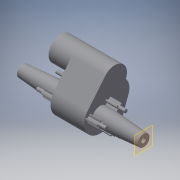
# Autodesk Inventor part: Back_Wheel_Drive
Saved by Autodesk Inventor 2019 (Build 230136000, 136)
## iProperties
Created: 2019-03-02
Part Number: Back_Wheel_Drive
Material: Generic
Document SubType Name: Modeling
Designer: alarr
Density: 1 g/cm^3
Appearance: Default
Author: alarr
Autodesk Inventor part; units mm, degrees
ref_plane "YZ Plane" through (0, 0, 0) normal (1, 0, 0) x (0, 1, 0)
ref_plane "XZ Plane" through (0, 0, 0) normal (0, 1, 0) x (-1, 0, 0)
ref_plane "XY Plane" through (0, 0, 0) normal (0, 0, 1) x (1, 0, 0)
sketch "Sketch1" plane through (0, 0, 0) normal (1, 0, 0) x (0, 1, 0)
  arc A0 (24.2941, -15.0442) -> (28.3956, -3.1971) centre (0, 0) ccw construction
  arc A1 (33.6079, -46.4865) -> (56.8822, -9.6036) centre (42.9735, -26.6116) ccw
  line L0 (18.0894, 22.1202) -> (56.8822, -9.6036)
  line L1 (-28.575, 0) -> (-28.575, -38.1)
  line L2 (-28.575, -38.1) -> (7.1559, -51.3254)
  arc A2 (-10.0486, -26.7499) -> (7.1559, -51.3254) centre (16.3035, -26.6116) ccw construction
  line L3 (42.9735, -26.6116) -> (16.3035, -26.6116) construction
  arc A3 (21.0025, -26.6116) -> (33.6079, -46.4865) centre (42.9735, -26.6116) ccw construction
  arc A4 (-10.0486, -26.7499) -> (24.2941, -15.0442) centre (0, 0) ccw construction
  arc A5 (28.3956, -3.1971) -> (18.0894, 22.1202) centre (0, 0) ccw construction
  arc A6 (18.0894, 22.1202) -> (-28.575, 0) centre (0, 0) ccw
  arc A7 (56.8822, -9.6036) -> (21.0025, -26.6116) centre (42.9735, -26.6116) ccw construction
  arc A8 (28.3956, -3.1971) -> (-10.0486, -26.7499) centre (16.3035, -26.6116) ccw construction
  arc A9 (-28.575, 0) -> (-10.0486, -26.7499) centre (0, 0) ccw construction
  arc A10 (7.1559, -51.3254) -> (33.6079, -46.4865) centre (16.3035, -26.6116) ccw
  arc A11 (33.6079, -46.4865) -> (28.3956, -3.1971) centre (16.3035, -26.6116) ccw construction
  dimension "d0" = 57.15
  dimension "d1" = 43.942
  dimension "d3" = 52.705
  dimension "d4" = 38.1
  dimension "d5" = 26.67
  constraints: 30 point on circle, 14 tangent, 12 centre point, 8 end point, 1 coincident, 1 equal length, 1 horizontal, 1 point on line, 1 vertical
  measures "d0" diameter of A0
  measures "d1" diameter of A1
  measures "d3" diameter of A2
  measures "d4" distance of L1.start L1.end
  measures "d5" distance of L3.start L3.end
extrude "Extrusion1" add sketch "Sketch1" along normal mid plane 60.579
sketch "Sketch2" plane through (30.2895, 0, 0) normal (1, 0, 0) x (0, 0, -1)
  circle A0 centre (0, 0) radius 14.605
  dimension "d8" = 29.21
  constraints: 1 centre point, 1 coincident
  measures "d8" diameter of A0
extrude "Extrusion2" add sketch "Sketch2" along normal blind 22.86
sketch "Sketch3" plane through (53.1495, 0, 0) normal (1, 0, 0) x (0, 0, -1)
  circle A0 centre (0, 0) radius 14.605 projected
  circle A1 centre (0, 0) radius 14.605
  constraints: 1 centre point, 1 coincident, 1 concentric
ref_plane "Work Plane1" through (109.0295, 0, 0) normal (1, 0, 0) x (0, 0, -1)
sketch "Sketch4" plane through (109.0295, 0, 0) normal (1, 0, 0) x (0, 0, -1)
  circle A0 centre (0, 0) radius 10.4775
  dimension "d12" = 20.955
  constraints: 1 centre point, 1 coincident
  measures "d12" diameter of A0
loft "Loft1" add profiles "Sketch3", "Sketch4"
sketch "Sketch5" plane through (109.0295, 0, 0) normal (1, 0, 0) x (0, 0, -1)
  circle A0 centre (0, 0) radius 4.191
  dimension "d17" = 8.382
  constraints: 1 centre point, 1 coincident
  measures "d17" diameter of A0
extrude "Extrusion3" cut sketch "Sketch5" against normal blind 12.7
sketch "Sketch6" plane through (30.2895, 0, 0) normal (1, 0, 0) x (0, 0, -1)
  circle A0 centre (0, 0) radius 19.9644 construction
  circle A1 centre (0, 0) radius 4.191 projected
  line L0 (0, 0) -> (0, -19.9644) construction
  line L1 (0, 0) -> (5.1672, -19.2841) construction
  circle A2 centre (5.1672, -19.2841) radius 2.9845
  circle A3 centre (0, 0) radius 14.605 construction
  line L2 (5.1672, -19.2841) -> (3.7801, -14.1073) construction
  circle A4 centre (0, 0) radius 4.191 projected
  circle A5 centre (0, 0) radius 14.605 construction
  dimension "d20" = 15
  dimension "d21" = 5.969
  dimension "d37" = 19.9644
  constraints: 6 end point, 3 coincident, 2 centre point, 2 point on circle, 1 point on line, 1 vertical, 5 other
  measures "d20" angle of L1 L0
  measures "d21" diameter of A2
  measures "d37" distance of L0.start L1.end
extrude "Extrusion4" add sketch "Sketch6" along normal blind 31.75 contours A2
sketch "Sketch7" plane through (30.2895, 0, 0) normal (1, 0, 0) x (0, 0, -1)
  circle A0 centre (0, 0) radius 14.605 projected
  circle A1 centre (5.1672, -19.2841) radius 2.9845 projected
  circle A2 centre (0, 0) radius 14.605
  circle A3 centre (5.1672, -19.2841) radius 2.9845
  line L0 (3.5151, -16.7986) -> (2.852, -14.3238)
  line L1 (5.3552, -16.3056) -> (4.692, -13.8308)
  line L2 (0, 0) -> (5.1672, -19.2841) construction
  line L3 (5.0236, -15.0682) -> (4.1036, -15.3147) construction
  line L4 (4.1036, -15.3147) -> (3.1835, -15.5612) construction
  dimension "d29" = 1.905
  constraints: 10 end point, 4 point on circle, 2 centre point, 2 coincident, 2 concentric, 2 midpoint, 2 parallel, 1 collinear, 1 perpendicular, 1 point on line
  measures "d29" distance between parallel lines of L1 L0
extrude "Extrusion5" add sketch "Sketch7" along normal blind 20.32 contours A0 L1 A1 L0
pattern_circular "Circular Pattern2" count 4 over 360 about axis through (30.2895, -19.2841, -5.1672) along (1, 0, 0) of "Extrusion5"
pattern_circular "Circular Pattern1" count 3 over 360 about axis through (109.0295, 0, 0) along (-1, 0, 0) of "Extrusion4", "Extrusion5", "Circular Pattern2"
mirror "Mirror1" about plane through (0, 0, 0) normal (1, 0, 0) of "Extrusion2", "Loft1", "Extrusion3", "Extrusion4", "Circular Pattern1"
sketch "Sketch8" plane through (-30.2895, 0, 0) normal (-1, 0, 0) x (0, 0, 1)
  arc A0 (-9.6036, 56.8822) -> (-46.4865, 33.6079) centre (-26.6116, 42.9735) ccw projected
  circle A1 centre (-26.6116, 42.9735) radius 21.971
  point P0 (0, 0)
  constraints: 1 centre point, 1 coincident, 1 concentric
extrude "Extrusion6" add sketch "Sketch8" along normal blind 36.83
body "Solid1"
